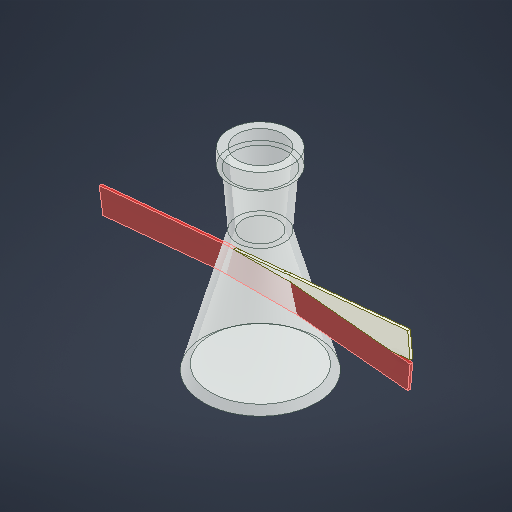
# Autodesk Inventor part: Симуляция преломления в конической колбе в зависимости от высоты
Saved by Autodesk Inventor 2026 (Build 300175000, 175)
## iProperties
Created: 2023-03-24
Part Number: Симуляция преломления в конической колбе в зависимости от высоты
Material: Типовые
Document SubType Name: Modeling
Designer: Admin
Density: 1 g/cm^3
Appearance: По умолчанию
Author: Admin
Autodesk Inventor part; units mm, degrees
ref_plane "YZ Plane" through (0, 0, 0) normal (1, 0, 0) x (0, 1, 0)
ref_plane "XZ Plane" through (0, 0, 0) normal (0, 1, 0) x (-1, 0, 0)
ref_plane "XY Plane" through (0, 0, 0) normal (0, 0, 1) x (1, 0, 0)
sketch "Эскиз1" plane through (0, 0, 0) normal (0, 0, 1) x (1, 0, 0)
  line L0 (-59.1772, 29.8139) -> (-11.5194, 34.2799)
  line L1 (-11.5194, 34.2799) -> (-9.4617, 34.2168)
  line L2 (-9.4617, 34.2168) -> (9.4617, 34.2168)
  line L3 (4.1486, 29.9467) -> (-11.5194, 34.2799) construction
  line L4 (5.2614, 30.1449) -> (-9.4617, 34.2168) construction
  line L5 (-8.6873, 29.1974) -> (9.4617, 34.2168) construction
  line L6 (9.4617, 34.2168) -> (11.5194, 34.2799)
  line L7 (11.5194, 34.2799) -> (55.9611, 30.1153)
  line L8 (11.5194, 34.2799) -> (-7.5026, 29.0191) construction
  line L9 (-57.7983, 20.9036) -> (-14.0859, 25)
  line L10 (-14.0859, 25) -> (-12.0283, 24.9369)
  line L11 (-12.0283, 24.9369) -> (12.0283, 24.9369)
  line L12 (12.0283, 24.9369) -> (14.0859, 25)
  line L13 (14.0859, 25) -> (55.1213, 21.1545)
  line L14 (1.508, 20.6873) -> (-14.0859, 25) construction
  line L15 (2.624, 20.8846) -> (-12.0283, 24.9369) construction
  line L16 (-5.9804, 19.9563) -> (12.0283, 24.9369) construction
  line L17 (-4.7984, 19.7773) -> (14.0859, 25) construction
  line L18 (0, 0) -> (21, 0)
  line L19 (21, 0) -> (8.5546, 45)
  line L20 (8.5546, 45) -> (10.0659, 65)
  line L21 (11.5, 65.5) -> (11.5, 71.5)
  line L22 (11.5, 71.5) -> (8.482, 71.5)
  line L23 (8.482, 71.5) -> (6.4795, 45)
  line L24 (6.4795, 45) -> (18.3718, 2)
  line L25 (18.3718, 2) -> (0, 2)
  line L26 (0, -7.6494) -> (0, -31.8354)
  line L27 (10.0659, 65) -> (11.5, 65.5)
  line L28 (0, 0) -> (-21, 0)
  line L29 (-21, 0) -> (-8.5546, 45)
  line L30 (-8.5546, 45) -> (-10.0659, 65)
  line L31 (-11.5, 65.5) -> (-11.5, 71.5)
  line L32 (-11.5, 71.5) -> (-8.482, 71.5)
  line L33 (-8.482, 71.5) -> (-6.4795, 45)
  line L34 (-6.4795, 45) -> (-18.3718, 2)
  line L35 (-18.3718, 2) -> (0, 2)
  line L36 (-10.0659, 65) -> (-11.5, 65.5)
  line L37 (55.0978, 40.3863) -> (10.9741, 36.2514)
  line L38 (55.9376, 31.4256) -> (13.411, 27.4404)
  line L39 (10.9741, 36.2514) -> (8.9837, 35.9454)
  line L40 (13.411, 27.4404) -> (11.4205, 27.1343)
  line L41 (11.4205, 27.1343) -> (-12.0283, 24.9369)
  line L42 (8.9837, 35.9454) -> (-9.4617, 34.2168)
  line L43 (55.9376, 31.4256) -> (55.0978, 40.3863)
  line L44 (55.1213, 21.1545) -> (55.9611, 30.1153)
  line L45 (-57.7983, 20.9036) -> (-59.1772, 29.8139)
  line L46 (0, 2) -> (0, 0)
  point P0 (48.958, 30.7715)
  dimension "Fall11" = 20.813
  dimension "d2" = 13.703
  dimension "Fall12" = 13.703
  dimension "d6" = 15.46
  dimension "Fall13" = 15.46
  dimension "d8" = 13.703
  dimension "Fall14" = 13.703
  dimension "d10" = 20.813
  dimension "Fall21" = 20.813
  dimension "d12" = 13.703
  dimension "Fall22" = 13.703
  dimension "d14" = 15.46
  dimension "Fall23" = 15.46
  dimension "d16" = 13.703
  dimension "Fall24" = 13.703
  dimension "d18" = 20.813
  dimension "d24" = 9
  dimension "d25" = 360
  dimension "d26" = 9.6283
  dimension "d27" = 2
  dimension "d28" = 2
  dimension "d29" = 21
  dimension "d30" = 12.959
  dimension "d31" = 16.964
  dimension "d32" = 11.5
  dimension "d33" = 0.5
  dimension "d34" = 6
  dimension "d35" = 20
  dimension "d36" = 45
  dimension "d37" = 25
  dimension "d38" = 69.187
  constraints: 94 end point, 13 point on line, 11 perpendicular, 8 symmetric about line, 3 parallel, 2 horizontal, 2 vertical, 1 coincident, 1 horizontal alignment, 1 vertical alignment
  measures "Fall11" angle of L0 L3
  measures "d2" angle of L1 L3
  measures "Fall12" angle of L4 L1
  measures "d6" angle of L2 L4
  measures "Fall13" angle of L2 L5
  measures "d8" angle of L6 L5
  measures "Fall14" angle of L6 L8
  measures "d10" angle of L8 L7
  measures "Fall21" angle of L9 L14
  measures "d12" angle of L10 L14
  measures "Fall22" angle of L10 L15
  measures "d14" angle of L11 L15
  measures "Fall23" angle of L11 L16
  measures "d16" angle of L12 L16
  measures "Fall24" angle of L17 L12
  measures "d18" angle of L17 L13
  measures "d24" distance between parallel lines of L0 L9
  measures "d26" distance of L6.end L12.end
  measures "d27" distance between parallel lines of L25 L18
  measures "d28" distance between parallel lines of L19 L24
  measures "d29" distance of L18.start L18.end
  measures "d30" diameter of L23.end L26
  measures "d31" diameter of L22.end L26
  measures "d32" distance from line of L18.start L21
  measures "d33" vertical distance of L21.start L20.end
  measures "d34" distance of L21.start L21.end
  measures "d35" vertical distance of L19.end L20.end
  measures "d36" vertical distance of L18.end L19.end
  measures "d37" distance from line of L9.end L28
  measures "d38" angle of L29 L9
revolve "Вращение1" add sketch "Эскиз1" angle 360 about axis through (0, -7.6494, 0) along (0, -1, 0) contours L24 L39 L19 L6 | L6 L19 L40 L24 | L24 L23 L22 L21 L27 L20 L19 L39 | L40 L19 L12 L24 | L12 L19 L18 L46 L25 L24
extrude "Выдавливание1" add sketch "Эскиз1" along normal mid plane 1 separate body contours L0 L29 L9 L45 | L1 L34 L10 L29 | L2 L24 L41 L34 | L6 L19 L40 L24 | L41 L24 L11 | L7 L38 L19 | L40 L19 L12 L24 | L7 L44 L13 L19 L38
extrude "Выдавливание2" add sketch "Эскиз1" along normal mid plane 1 separate body contours L42 L24 L2 | L24 L39 L19 L6 | L19 L37 L43 L38 L7
equation "\"n2\" = 1.5"
equation "\"n3\" = 1.333"
